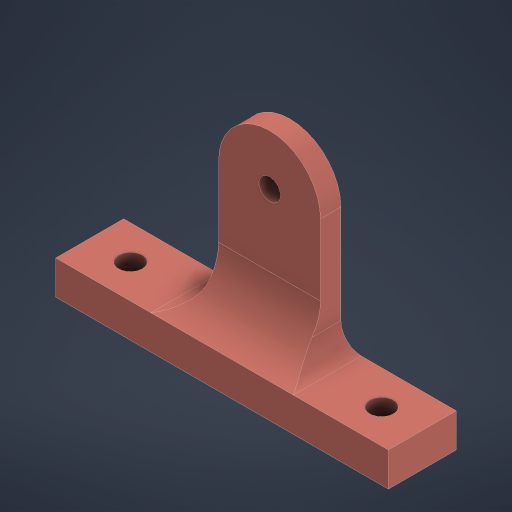
# Autodesk Inventor part: soporte_base
Saved by Autodesk Inventor 2023.1 (Build 271208000, 208)
## iProperties
Created: 2022-11-06
Part Number: soporte_base
Material: Generic
Document SubType Name: Modeling
Designer: amtat
Density: 1 g/cm^3
Appearance: Default
Author: amtat
Autodesk Inventor part; units mm, degrees
ref_plane "YZ Plane" through (0, 0, 0) normal (1, 0, 0) x (0, 1, 0)
ref_plane "XZ Plane" through (0, 0, 0) normal (0, 1, 0) x (-1, 0, 0)
ref_plane "XY Plane" through (0, 0, 0) normal (0, 0, 1) x (1, 0, 0)
sketch "Sketch1" plane through (0, 0, 0) normal (0, 0, 1) x (1, 0, 0)
  line L0 (0, 0) -> (0, 22.5)
  circle A0 centre (0, 22.5) radius 7.5
  line L1 (7.5, 22.5) -> (7.5, 0)
  line L2 (7.5, 0) -> (-7.5, 0)
  line L3 (-7.5, 0) -> (-7.5, 22.5)
  circle A1 centre (0, 22.5) radius 1.6
  line L4 (7.5, 0) -> (24.5, 0)
  line L5 (-7.5, 0) -> (-24.5, 0)
  line L6 (24.5, 0) -> (24.5, 5)
  line L7 (24.5, 5) -> (7.5, 5)
  line L8 (-24.5, 0) -> (-24.5, 5)
  line L9 (-24.5, 5) -> (-7.5, 5)
  dimension "d0" = 22.5
  dimension "d2" = 15
  dimension "d3" = 15
  dimension "d4" = 3.2
  dimension "d5" = 17
  dimension "d6" = 17
  dimension "d7" = 5
  dimension "d8" = 5
  constraints: 20 end point, 4 point on line, 3 vertical, 2 centre point, 2 horizontal, 2 perpendicular, 2 point on circle, 1 coincident, 1 tangent
  measures "d0" distance of L0.start L0.end
  measures "d2" diameter of A0
  measures "d3" distance of L1.end L2.end
  measures "d4" diameter of A1
  measures "d5" distance of L1.end L4.end
  measures "d6" distance of L2.end L5.end
  measures "d7" distance of L4.end L6.end
  measures "d8" distance of L5.end L8.end
extrude "Extrusion1" add sketch "Sketch1" along normal blind 3
sketch "Sketch2" plane through (0, 0, 3) normal (0, 0, 1) x (1, 0, 0)
  line L0 (-7.5, 22.5) -> (-7.5, 5) projected
  line L1 (-7.5, 5) -> (-24.5, 5) projected
  line L2 (-24.5, 5) -> (-24.5, 0) projected
  line L3 (-24.5, 0) -> (24.5, 0) projected
  line L4 (24.5, 0) -> (24.5, 5) projected
  line L5 (24.5, 5) -> (7.5, 5) projected
  line L6 (7.5, 5) -> (7.5, 22.5) projected
  arc A0 (7.5, 22.5) -> (-7.5, 22.5) centre (0, 22.5) ccw projected
  circle A1 centre (0, 22.5) radius 1.6 projected
  line L7 (-7.5, 22.5) -> (-7.5, 5) projected
  line L8 (24.5, 5) -> (7.5, 5) projected
  line L9 (-7.5, 5) -> (7.5, 5)
  point P0 (0, 0)
  constraints: 2 end point, 1 horizontal
extrude "Extrusion2" add sketch "Sketch2" along normal blind 7 contours L9 L5 L4 L3 L2 L1
sketch "Sketch3" plane through (-24.5, 5, 0) normal (0, 1, 0) x (1, 0, 0)
  line L0 (17, 0) -> (0, 0) projected
  line L1 (0, 0) -> (0, -10) projected
  line L2 (49, -10) -> (0, -10) projected
  line L3 (49, 0) -> (49, -10) projected
  line L4 (49, 0) -> (32, 0) projected
  line L5 (32, 0) -> (32, -3) projected
  line L6 (17, -3) -> (32, -3) projected
  line L7 (17, 0) -> (17, -3) projected
  line L8 (0, 0) -> (0, -5)
  line L9 (0, 0) -> (0, -10) projected
  line L10 (0, -5) -> (6, -5)
  circle A0 centre (6, -5) radius 1.75
  line L11 (49, 0) -> (32, 0) projected
  line L12 (49, 0) -> (49, -5)
  line L13 (49, 0) -> (49, -10) projected
  line L14 (49, -5) -> (43, -5)
  circle A1 centre (43, -5) radius 1.75
  point P0 (24.5, 0)
  dimension "d13" = 5
  dimension "d14" = 6
  dimension "d15" = 3.5
  dimension "d16" = 5
  dimension "d17" = 6
  dimension "d18" = 3.5
  constraints: 8 end point, 2 centre point, 2 coincident, 2 midpoint, 2 perpendicular
  measures "d13" distance of L0.end L8.end
  measures "d14" distance of L8.end L10.end
  measures "d15" diameter of A0
  measures "d16" distance of L3.start L12.end
  measures "d17" distance of L12.end L14.end
  measures "d18" diameter of A1
extrude "Extrusion3" cut sketch "Sketch3" against normal blind 7 contours A0 | A1
fillet "Fillet1" radius 3 2 edges at (-7.5, 5, 1.5) (7.5, 5, 1.5)
fillet "Fillet2" radius 7 3 edges at (9, 5, 3) (0, 5, 3) (-9, 5, 3)
body "Solid1"
